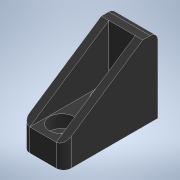
# Autodesk Inventor part: 27_Switch_Holder_X
Saved by Autodesk Inventor 2022.2 (Build 262287010, 287A)
## iProperties
Created: 2022-05-06
Part Number: 27_Switch_Holder_X
Material: PET-Kunststoff
Document SubType Name: Modeling
Designer: MXBD
Density: 1.541 g/cm^3
Appearance: Gummi - Schwarz
Author: MXBD
Autodesk Inventor part; units mm, degrees
ref_plane "YZ Plane" through (0, 0, 0) normal (1, 0, 0) x (0, 1, 0)
ref_plane "XZ Plane" through (0, 0, 0) normal (0, 1, 0) x (-1, 0, 0)
ref_plane "XY Plane" through (0, 0, 0) normal (0, 0, 1) x (1, 0, 0)
sketch "Skizze1" plane through (0, 0, 0) normal (1, 0, 0) x (0, 1, 0)
  line L0 (0, 30) -> (0, -5) projected
  line L1 (-4, 0) -> (24, 0) projected
  line L2 (0, 25) -> (0, 0)
  line L3 (0, 0) -> (20, 0)
  line L4 (20, 0) -> (20, 4)
  line L5 (20, 4) -> (6, 4)
  line L6 (6, 4) -> (6, 25)
  line L7 (6, 25) -> (0, 25)
  dimension "d0" = 20
  dimension "d1" = 25
  dimension "d2" = 4
  dimension "d3" = 6
  constraints: 12 end point, 4 perpendicular, 2 point on line, 1 vertical
  measures "d0" distance between parallel lines of L2 L4
  measures "d1" distance between parallel lines of L3 L7
  measures "d2" distance between parallel lines of L3 L5
  measures "d3" distance between parallel lines of L2 L6
extrude "Extrusion1" add sketch "Skizze1" along normal mid plane 11
sketch "Skizze2" plane through (-5.5, 6, 25) normal (0, 1, 0) x (1, 0, 0)
  line L0 (5.5, 30) -> (5.5, -5) projected
  line L1 (11, 0) -> (0, 0) projected
  point P0 (5.5, 25)
  point P1 (5.5, 5)
  point P2 (5.5, 17)
  dimension "d6" = 5
  dimension "d14" = 12
  constraints: 2 point on line
  measures "d6" distance from line of L1 point (5.5, 5)
  measures "d14" distance of point (5.5, 17) point (5.5, 5)
hole "Bohrung1" at (0, 6, 20) at (0, 6, 8) direction (0, -1, 0) diameter 3.4 end through all counterbore diameter 6.5 counterbore depth 3.4 clearance for "Inbusschraube ISO 4762" size "M3" standard "ISO"
sketch "Skizze3" plane through (0, 0, 0) normal (1, 0, 0) x (0, 1, 0)
  line L0 (20, 4) -> (6, 4) projected
  line L1 (6, 25) -> (0, 25) projected
  line L2 (20, 4) -> (6, 25)
  line L3 (6, 25) -> (6, 4)
  line L4 (6, 4) -> (20, 4)
  point P0 (0, 0)
  point P1 (6, 4)
  constraints: 6 end point, 2 perpendicular
extrude "Extrusion2" add sketch "Skizze3" against normal blind 2 from surface at 5.5
mirror "Spiegeln1" about plane through (0, 0, 0) normal (1, 0, 0) of "Extrusion2"
fillet "Rundung2" radius 2 3 edges at (0, 20, 0) (5.5, 3, 25) (-5.5, 3, 25)
